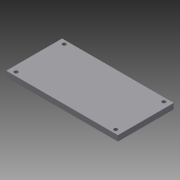
# Autodesk Inventor part: electronics
Saved by Autodesk Inventor 2014 (Build 180170000, 170)
## iProperties
Created: 2013-07-26
Part Number: electronics
Material: Generic
Document SubType Name: Modeling
Designer: employee
Density: 1 g/cm^3
Mass: 25.6248 g
Surface Area: 119.876 cm^2
Volume: 25.6248 cm^3
Appearance: Smooth - Dark Forest Green
Author: employee
Autodesk Inventor part; units mm, degrees
ref_plane "YZ Plane" through (0, 0, 0) normal (1, 0, 0) x (0, 1, 0)
ref_plane "XZ Plane" through (0, 0, 0) normal (0, 1, 0) x (-1, 0, 0)
ref_plane "XY Plane" through (0, 0, 0) normal (0, 0, 1) x (1, 0, 0)
sketch "Sketch1" plane through (0, 0, 0) normal (0, 0, 1) x (1, 0, 0)
  line L0 (-50.8, -25.4) -> (50.8, -25.4)
  line L1 (50.8, -25.4) -> (50.8, 25.4)
  line L2 (50.8, 25.4) -> (-50.8, 25.4)
  line L3 (-50.8, 25.4) -> (-50.8, -25.4)
  point P0 (0, 0)
  point P1 (0, 25.4)
  point P2 (50.8, 0)
  dimension "d12" = 90
  dimension "d0" = 50.8
  dimension "d2" = 101.6
  constraints: 8 end point, 2 midpoint, 2 parallel, 1 horizontal, 1 horizontal alignment, 1 perpendicular, 1 vertical alignment
  measures "d0" distance of L0.end L1.end
  measures "d2" distance of L0.start L0.end
extrude "Extrusion1" add sketch "Sketch1" along normal blind 5
sketch "Sketch2" plane through (0, 0, 5) normal (0, 0, 1) x (1, 0, 0)
  line L0 (50.8, -25.4) -> (50.8, 25.4) projected
  line L1 (50.8, 25.4) -> (-50.8, 25.4) projected
  line L2 (-45.339, 21.9075) -> (45.339, 21.9075)
  line L3 (45.339, 21.9075) -> (45.339, -21.9075)
  line L4 (45.339, -21.9075) -> (-45.339, -21.9075)
  line L5 (-45.339, -21.9075) -> (-45.339, 21.9075)
  point P0 (45.339, 0)
  point P1 (50.8, 0)
  point P2 (0, 21.9075)
  point P3 (0, 25.4)
  dimension "d5" = 43.815
  dimension "d7" = 90.678
  constraints: 8 end point, 4 midpoint, 2 parallel, 1 horizontal, 1 horizontal alignment, 1 perpendicular, 1 vertical alignment
  measures "d5" distance of L2.end L3.end
  measures "d7" distance of L2.start L2.end
hole "Hole1" at (-45.339, 21.9075, 5) at (45.339, 21.9075, 5) at (45.339, -21.9075, 5) at (-45.339, -21.9075, 5) direction (0, 0, -1) diameter 3.4 end through all clearance for "Socket Head Cap Screw" size "M3" standard "Ansi Metric M Profile"
body "Solid1"
